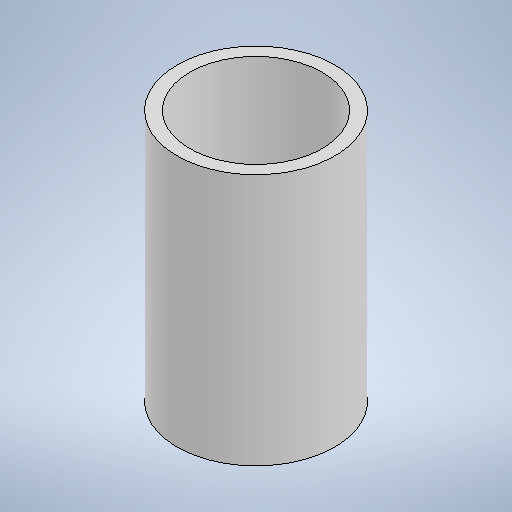
# Autodesk Inventor part: M3Adapter
Saved by Autodesk Inventor 2026 (Build 300175050, 175E)
## iProperties
Created: 2025-12-26
Part Number: M3Adapter
Material: Generic
Document SubType Name: Modeling
Designer: Nicholas M
Density: 1 g/cm^3
Appearance: Default
Author: Nicholas M
Autodesk Inventor part; units mm, degrees
ref_plane "YZ Plane" through (0, 0, 0) normal (1, 0, 0) x (0, 1, 0)
ref_plane "XZ Plane" through (0, 0, 0) normal (0, 1, 0) x (-1, 0, 0)
ref_plane "XY Plane" through (0, 0, 0) normal (0, 0, 1) x (1, 0, 0)
sketch "Sketch1" plane through (0, 0, 0) normal (0, 1, 0) x (-1, 0, 0)
  circle A0 centre (0, 0) radius 1.575
  circle A1 centre (0, 0) radius 1.875
  dimension "d0" = 3.15
  dimension "d1" = 3.75
  constraints: 2 centre point, 2 coincident
  measures "d0" diameter of A0
  measures "d1" diameter of A1
extrude "Extrusion1" add sketch "Sketch1" along normal blind 6
body "Solid1"
